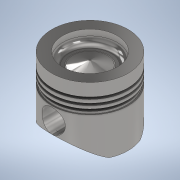
# Autodesk Inventor part: piston
Saved by Autodesk Inventor 2021 (Build 250183000, 183)
## iProperties
Created: 2020-11-23
Part Number: piston
Material: Сталь, высокопрочная, низколегированная
Document SubType Name: Modeling
Designer: panda
Mass: 1909.1 g
Surface Area: 573.952 cm^2
Volume: 243.197 cm^3
Density: 7.85 g/cm^3
Appearance: Сталь — полированная
Author: panda
Autodesk Inventor part; units mm, degrees
ref_plane "YZ Plane" through (0, 0, 0) normal (1, 0, 0) x (0, 1, 0)
ref_plane "XZ Plane" through (0, 0, 0) normal (0, 1, 0) x (-1, 0, 0)
sketch "Эскиз1" plane through (0, 0, 0) normal (0, 0, 1) x (1, 0, 0)
  line L0 (32.55, 0) -> (45.55, 0)
  line L1 (45.55, 0) -> (45.55, -80)
  line L2 (45.55, -80) -> (0, -80)
  line L3 (0, -80) -> (0, -9)
  line L4 (45.55, 0) -> (32.55, 0)
  line L5 (32.55, 0) -> (32.55, -7)
  arc A0 (25.05, -14.5) -> (32.55, -7) centre (25.05, -7) ccw
  line L6 (25.05, -7) -> (25.05, -14.5) construction
  line L7 (25.05, -7) -> (32.55, -7) construction
  line L8 (0, -9) -> (22.6563, -9) construction
  line L9 (21.7112, -14.5) -> (25.05, -14.5)
  arc A1 (20.4171, -14.3296) -> (21.7112, -14.5) centre (21.7112, -9.5) ccw
  line L10 (45.55, -15) -> (39.05, -15)
  line L11 (39.05, -15) -> (39.05, -17.5)
  line L12 (39.05, -17.5) -> (45.55, -17.5)
  line L13 (45.55, -21.5) -> (39.55, -21.5)
  line L14 (39.55, -21.5) -> (39.55, -24)
  line L15 (39.55, -24) -> (45.55, -24)
  line L16 (45.55, -27.5) -> (39.55, -27.5)
  line L17 (39.55, -27.5) -> (39.55, -31)
  line L18 (39.55, -31) -> (44.05, -31)
  line L19 (44.05, -31) -> (44.05, -33.5)
  line L20 (44.05, -33.5) -> (45.55, -33.5)
  line L21 (20.4171, -14.3296) -> (1.0353, -9.1363)
  arc A2 (1.0353, -9.1363) -> (0, -9) centre (0, -13) ccw
  line L22 (35.0546, -24) -> (35.0546, -19)
  line L23 (28.9454, -19) -> (28.9454, -24)
  arc A3 (35.0546, -19) -> (28.9454, -19) centre (32, -19) ccw
  line L24 (28.9454, -21.5) -> (35.0546, -21.5)
  arc A4 (28.9454, -24) -> (35.0546, -24) centre (32, -24) ccw
  point P0 (0, 0)
  point P1 (0.5266, -9)
  dimension "d0" = 80
  dimension "d1" = 45.55
  dimension "d2" = 13
  dimension "d3" = 7
  dimension "d5" = 7.5
  dimension "d7" = 9
  dimension "d8" = 5
  dimension "d9" = 180
  dimension "d10" = 2.5
  dimension "d11" = 6.5
  dimension "d12" = 2.5
  dimension "d13" = 3.5
  dimension "d14" = 4
  dimension "d15" = 15
  dimension "d17" = 2.5
  dimension "d18" = 1.5
  dimension "d20" = 6
  dimension "d21" = 6
  dimension "d22" = 3.5
  dimension "d34" = 4
  dimension "d36" = 15
  dimension "d38" = 5
  constraints: 50 end point, 11 perpendicular, 10 point on circle, 10 point on line, 5 centre point, 5 horizontal, 5 tangent, 3 horizontal alignment, 2 midpoint, 2 vertical, 1 parallel, 1 symmetric about line, 1 vertical alignment, 1 other
  measures "d0" distance of L0.end L1.end
  measures "d1" distance of point (0, 0) L0.end
  measures "d2" distance of L0.start L0.end
  measures "d3" distance of L0.start L5.end
  measures "d5" radius of A0
  measures "d7" distance from line of L3.end L0
  measures "d8" radius of A1
  measures "d9" angle of L5 L6
  measures "d10" distance of L10.end L11.end
  measures "d11" distance of L10.start L10.end
  measures "d12" distance of L13.end L14.end
  measures "d13" distance of L16.end L17.end
  measures "d14" distance of L13.start L12.end
  measures "d15" distance of L10.start L0.end
  measures "d17" distance of L18.end L19.end
  measures "d18" distance of L19.end L20.end
  measures "d20" distance of L13.start L13.end
  measures "d21" distance of L16.start L16.end
  measures "d22" distance of L16.start L15.end
  measures "d34" radius of A2
  measures "d36" angle of L8 L21
  measures "d38" distance of L22.start L22.end
revolve "Вращение1" add sketch "Эскиз1" angle 360 about axis through (0, -80, 0) along (0, 1, 0) contours L0 L1 L10 L11 L12 L13 L14 L15 L16 L17 L18 L19 L20 L2 L3 A2 L21 A1 L9 A0 L5 | A4 L23 L24 L22 | L24 L23 A3 L22
sketch "Эскиз2" plane through (0, 0, 0) normal (0, 0, 1) x (1, 0, 0)
  line L0 (-39.05, -15) -> (39.05, -15) projected
  line L1 (-39.55, -27.5) -> (39.55, -27.5) projected
  line L2 (0, -63.05) -> (-39.05, -63.05) construction
  line L3 (0, -63.05) -> (0, -27.5) construction
  line L4 (-39.05, -63.05) -> (-39.05, -88.4804)
  line L5 (-45.55, -80) -> (45.55, -80) projected
  line L6 (-39.05, -88.4804) -> (0, -88.4804)
  line L7 (0, -88.4804) -> (0, -27.5)
  line L8 (0, -27.5) -> (0, -24)
  line L9 (-39.55, -24) -> (39.55, -24) projected
  arc A0 (0, -24) -> (-39.05, -63.05) centre (0, -63.05) ccw
  point P0 (0, 0)
  dimension "d23" = 90
  constraints: 12 end point, 3 perpendicular, 2 midpoint, 2 point on circle, 2 vertical alignment, 1 centre point, 1 coincident
  measures "d23" angle of L3 L2
revolve "Вращение2" cut sketch "Эскиз2" angle 360 about axis through (0, -63.05, 0) along (0, 1, 0)
sketch "Эскиз3" plane through (0, 0, 0) normal (0, 0, 1) x (1, 0, 0)
  circle A0 centre (0, -122.4513) radius 59.4013
  line L0 (-45.55, -80) -> (45.55, -80) projected
  line L1 (-41.55, -80) -> (41.55, -80)
  line L2 (-39.05, -63.05) -> (39.05, -63.05) projected
  point P0 (0, 0)
  dimension "d25" = 4
  constraints: 2 end point, 2 point on circle, 2 point on line, 1 centre point, 1 collinear, 1 tangent, 1 vertical alignment
  measures "d25" distance of L0.end L1.end
extrude "Выдавливание1" cut sketch "Эскиз3" along normal through all both and the other way through all
ref_plane "РабПлоскость1" through (0, 0, 39.05) normal (0, 0, 1) x (1, 0, 0)
sketch "Эскиз4" plane through (0, 0, 39.05) normal (0, 0, 1) x (1, 0, 0)
  circle A0 centre (0, -49.0033) radius 17.5467
  point P0 (0, 0)
  constraints: 1 centre point
extrude "Выдавливание2" add sketch "Эскиз4" against normal blind 20
mirror "Зеркальное отражение1" about plane through (0, 0, 0) normal (0, 0, 1) of "Выдавливание2"
sketch "Эскиз5" plane through (0, -49.0033, -19.05) normal (0, 0, 1) x (1, 0, 0)
  arc A0 (17.5467, 0) -> (17.5467, 0) centre (0, 0) ccw projected
  circle A1 centre (0, 0) radius 14
  point P0 (0, 49.0033)
  dimension "d31" = 28
  constraints: 1 centre point, 1 coincident
  measures "d31" diameter of A1
extrude "Выдавливание3" cut sketch "Эскиз5" along normal through all both and the other way through all contours A1
